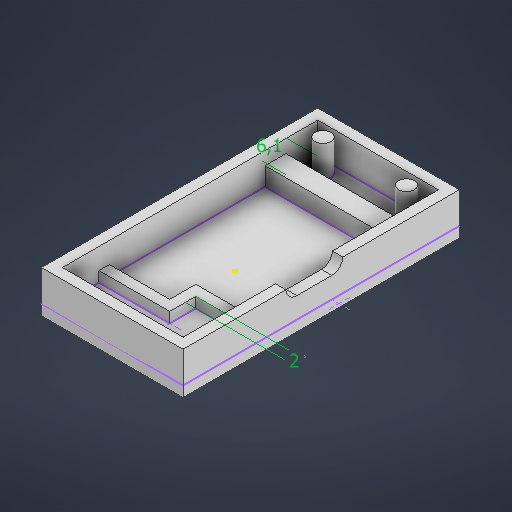
# Autodesk Inventor part: base
Saved by Autodesk Inventor 2026.2 (Build 302298010, 298A)
## iProperties
Created: 2026-05-20
Part Number: base
Material: Generic
Document SubType Name: Modeling
Designer: anton
Density: 1 g/cm^3
Appearance: Default
Author: anton
Autodesk Inventor part; units mm, degrees
ref_plane "YZ Plane" through (0, 0, 0) normal (1, 0, 0) x (0, 1, 0)
ref_plane "XZ Plane" through (0, 0, 0) normal (0, 1, 0) x (-1, 0, 0)
ref_plane "XY Plane" through (0, 0, 0) normal (0, 0, 1) x (1, 0, 0)
sketch "Sketch1" plane through (0, 0, 0) normal (0, 1, 0) x (-1, 0, 0)
  circle A0 centre (-8.0963, -24.7317) radius 1.5
  circle A1 centre (7.9037, -24.7317) radius 1.5
  line L0 (-11.8963, -27.0317) -> (11.2037, -27.0317)
  line L1 (11.2037, 21.8683) -> (-11.8963, 21.8683)
  line L2 (-0.3463, 7.8683) -> (-0.3463, 9.8683)
  line L3 (-2.3463, 9.8683) -> (-11.8963, 9.8683)
  line L4 (-13.8963, -29.0317) -> (13.2037, -29.0317)
  line L5 (13.2037, -29.0317) -> (13.2037, 23.8683)
  line L6 (13.2037, 23.8683) -> (-13.8963, 23.8683)
  line L7 (-13.8963, 23.8683) -> (-13.8963, -29.0317)
  line L8 (-0.3463, 7.8683) -> (-11.8963, 7.8683)
  line L9 (-11.8963, 21.8683) -> (-11.8963, 7.8683)
  line L10 (11.2037, 12.8683) -> (-0.3463, 12.8683)
  line L11 (-0.3463, 9.8683) -> (-0.3463, 12.8683)
  line L12 (-2.3463, 14.8683) -> (-2.3463, 9.8683)
  line L13 (-2.3463, 14.8683) -> (11.2037, 14.8683)
  line L14 (11.2037, -16.9317) -> (-11.8963, -16.9317)
  line L15 (-11.8963, -20.9317) -> (11.2037, -20.9317)
  line L16 (-11.8963, 7.8683) -> (-11.8963, -20.9317)
  line L17 (-11.8963, -20.9317) -> (-11.8963, -27.0317)
  line L18 (11.2037, -27.0317) -> (11.2037, 21.8683)
  point P0 (0, 0)
  point P1 (-15.2463, -4.6317)
  dimension "d0" = 2
  dimension "d12" = 6.1
  constraints: 38 end point, 9 perpendicular, 4 parallel, 2 centre point, 2 point on line, 2 vertical, 1 coincident, 1 horizontal
  measures "d0" distance of L2.start L2.end
  measures "d12" distance between parallel lines of L0 L15
extrude "Extrusion1" add sketch "Sketch1" against normal blind 2 contours A0 | A1 | L17 L15 L18 L0 | L16 L14 L18 L15 | L16 L8 L2 L11 L10 L18 L14 | L9 L3 L12 L13 L18 L10 L11 L2 L8 | L9 L1 L18 L13 L12 L3 | L7 L6 L5 L4
extrude "Extrusion2" add sketch "Sketch1" along normal blind 6
extrude "Extrusion3" add sketch "Sketch1" along normal blind 2 contours L9 L3 L12 L13 L18 L10 L11 L2 L8
extrude "Extrusion4" add sketch "Sketch1" along normal blind 3.5 contours L16 L14 L18 L15
sketch "Sketch3" plane through (13.8963, -2, 23.8683) normal (1, 0, 0) x (0, 0, -1)
  arc A0 (30.6, 9.1) -> (28.5, 11.2) centre (28.5, 9.1) ccw
  arc A1 (21.8, 11.2) -> (19.7, 9.1) centre (21.8, 9.1) ccw
  line L0 (20.7, 8.1) -> (20.7, 9.1)
  line L1 (20.7, 8.1) -> (20.7, 9.1)
  line L2 (20.7, 9.1) -> (20.7, 8.1)
  arc A2 (21.8, 10.2) -> (20.7, 9.1) centre (21.8, 9.1) ccw
  line L3 (0, 0) -> (0, 8)
  line L4 (29.6, 9.1) -> (29.6, 8.1)
  line L5 (29.6, 8.1) -> (29.6, 9.1)
  line L6 (28.5, 10.2) -> (21.8, 10.2)
  arc A3 (29.6, 9.1) -> (28.5, 10.2) centre (28.5, 9.1) ccw
  line L7 (30.6, 8.1) -> (30.6, 9.1)
  line L8 (29.6, 8.1) -> (29.6, 9.1)
  arc A4 (28.5, 6) -> (30.6, 8.1) centre (28.5, 8.1) ccw
  line L9 (28.5, 11.2) -> (21.8, 11.2)
  line L10 (21.8, 10.2) -> (28.5, 10.2)
  line L11 (28.5, 10.2) -> (21.8, 10.2)
  line L12 (21.8, 7) -> (28.5, 7)
  line L13 (28.5, 7) -> (21.8, 7)
  line L14 (21.8, 6) -> (28.5, 6)
  line L15 (19.7, 9.1) -> (19.7, 8.1)
  arc A5 (20.7, 8.1) -> (21.8, 7) centre (21.8, 8.1) ccw
  arc A6 (19.7, 8.1) -> (21.8, 6) centre (21.8, 8.1) ccw
  line L16 (52.9, 8) -> (52.9, 0)
  line L17 (0, 8) -> (52.9, 8)
  line L18 (52.9, 0) -> (0, 0)
  arc A7 (28.5, 7) -> (29.6, 8.1) centre (28.5, 8.1) ccw
  point P0 (23.8683, 2)
  point P1 (29.0317, 2)
  point P2 (20.7, 10.2)
  point P3 (29.6, 7)
  point P4 (30.5976, 8)
  point P5 (19.7024, 8)
  dimension "d21" = 1.1
  dimension "d22" = 1
  constraints: 38 end point, 16 point on circle, 8 centre point, 6 point on line
  measures "d21" radius of A2
  measures "d22" radial gap between concentric circles of A2 A1
extrude "Extrusion6" cut sketch "Sketch3" against normal blind 6 contours A4 L14 A6 L17 A5 L12 A7 | A7 L12 A5 L17
body "Solid1"
